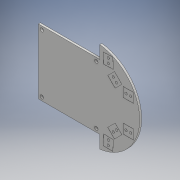
# Autodesk Inventor part: PCB_final
Saved by Autodesk Inventor 2017 (Build 210142000, 142)
## iProperties
Created: 2016-07-30
Part Number: PCB_final
Material: Generic
Document SubType Name: Modeling
Designer: ANDRES
Density: 1 g/cm^3
Appearance: Default
Author: ANDRES
Autodesk Inventor part; units mm, degrees
ref_plane "YZ Plane" through (0, 0, 0) normal (1, 0, 0) x (0, 1, 0)
ref_plane "XZ Plane" through (0, 0, 0) normal (0, 1, 0) x (-1, 0, 0)
ref_plane "XY Plane" through (0, 0, 0) normal (0, 0, 1) x (1, 0, 0)
sketch "Sketch1" plane through (0, 0, 0) normal (0, 1, 0) x (-1, 0, 0)
  circle A0 centre (-24.5, -25) radius 1.5
  circle A1 centre (-24.5, 25) radius 1.5
  circle A2 centre (22.5, 25) radius 1.5
  circle A3 centre (22.5, -25) radius 1.5
  line L0 (-27.5, -28) -> (-8, -28)
  line L1 (-8, -28) -> (-8, -25) construction
  line L2 (6, -25) -> (6, -28) construction
  line L3 (6, -28) -> (25.5, -28)
  line L4 (25.5, -28) -> (25.5, 28)
  line L5 (25.5, 28) -> (6, 28)
  line L6 (-8, 28) -> (-27.5, 28)
  line L7 (-27.5, 28) -> (-27.5, 39.1)
  arc A4 (-27.5, 39.1) -> (-27.5, -39.1) centre (-22.3277, 0) ccw
  line L8 (-27.5, -39.1) -> (-27.5, -28)
  line L9 (-8, 28) -> (6, 28)
  line L10 (-8, -25) -> (-8, 28) construction
  line L11 (6, -25) -> (6, 28) construction
  line L12 (-8, -28) -> (6, -28)
  line L13 (22.75, 28) -> (-24.75, 28) construction
  line L14 (-24.75, 22) -> (22.75, 22) construction
  line L15 (25.5, -22) -> (-24.75, -22) construction
  line L16 (-24.75, -28) -> (22.75, -28) construction
  line L17 (-8, 28) -> (-27.5, 28) construction
  line L18 (-27.5, 28) -> (-27.5, 39.1) construction
  arc A5 (-27.5, 39.1) -> (-27.5, -39.1) centre (-22.3277, 0) ccw construction
  circle A6 centre (-38.9568, 20.5358) radius 1
  line L19 (-40.0897, 25.2111) -> (-34.2841, 19.3919)
  line L20 (-46.4612, 18.8546) -> (-40.0897, 25.2111)
  circle A7 centre (-41.7885, 17.7107) radius 1
  line L21 (-46.4612, 18.8546) -> (-40.6556, 13.0354)
  line L22 (-34.2841, 19.3919) -> (-40.6556, 13.0354)
  line L23 (-39.9854, 35.3107) -> (-39.9038, 35.3078) construction
  circle A8 centre (-34.6947, 32.6244) radius 1
  line L24 (-39.0291, 26.2718) -> (-38.7163, 35.2301)
  circle A9 centre (-34.8343, 28.6268) radius 1
  line L25 (-39.0291, 26.2718) -> (-30.8141, 25.9849)
  line L26 (-30.5, 34.9794) -> (-30.8141, 25.9849)
  circle A10 centre (-50.0144, 13.6765) radius 1
  line L27 (-47.5144, 9.5665) -> (-47.5144, 17.7865)
  circle A11 centre (-54.0144, 13.6765) radius 1
  line L28 (-56.5144, 17.7865) -> (-47.5144, 17.7865)
  line L29 (-56.5144, 9.5665) -> (-56.5144, 17.7865)
  line L30 (-47.5144, 9.5665) -> (-56.5144, 9.5665)
  line L31 (-39.0291, 26.2718) -> (-67.0612, -1.7603) construction
  line L32 (-39.0291, 26.2718) -> (0.6143, 26.2718) construction
  line L33 (-38.7163, 35.2301) -> (-30.5, 34.9794)
  line L34 (-27.5, -28) -> (-27.5, -22) construction
  line L35 (-27.5, -22) -> (-24.75, -22) construction
  line L36 (-27.5, 28) -> (-27.5, 22) construction
  line L37 (-24.75, 22) -> (-27.5, 22) construction
  line L38 (-27.5, 22) -> (-27.5, 28) construction
  line L39 (-27.5, -22) -> (-27.5, -28) construction
  point P0 (0, 0)
  point P1 (0, 0)
  point P2 (-1, 28)
  point P3 (-1, -22)
  point P4 (-1, -28)
  point P5 (0, 0)
  point P6 (4.5, 0)
  dimension "d0" = 47.5
  dimension "d1" = 6
  dimension "d3" = 47.5
  dimension "d4" = 6
  dimension "d8" = 39.4406
  dimension "d9" = 5.1723
  dimension "d10" = 3
  dimension "d11" = 3
  dimension "d12" = 3
  dimension "d13" = 3
  dimension "d14" = 2
  dimension "d15" = 2
  dimension "d16" = 135
  dimension "d17" = 178
  dimension "d18" = 180
  dimension "d19" = 1.5
  dimension "d20" = 1.5
  dimension "d21" = 1.7282
  dimension "d22" = 8.22
  dimension "d23" = 9
  dimension "d24" = 2
  dimension "d25" = 2
  dimension "d26" = 2.5
  dimension "d27" = 4.11
  dimension "d28" = 4.11
  dimension "d29" = 2.5
  dimension "d30" = 8.22
  dimension "d31" = 2.5
  dimension "d32" = 9
  dimension "d33" = 2.5
  dimension "d34" = 4.11
  dimension "d35" = 4.11
  dimension "d36" = 9
  dimension "d37" = 8.22
  dimension "d38" = 4.11
  dimension "d39" = 2.5
  dimension "d40" = 2.5
  dimension "d41" = 4.11
  dimension "d42" = 3
  dimension "d58" = 3
  dimension "d59" = 53
  dimension "d60" = 3
  dimension "d61" = 3
  dimension "d62" = 3
  constraints: 80 end point, 12 centre point, 7 horizontal, 6 perpendicular, 5 point on circle, 5 point on line, 4 midpoint, 4 parallel, 2 collinear, 1 equal length, 1 vertical
  measures "d0" distance of L14.end L14.start
  measures "d1" distance of L14.start L13.end
  measures "d3" distance of L16.end L16.start
  measures "d4" distance of L16.start L15.end
  measures "d8" radius of A4
  measures "d9" distance from line of L8 A4.centre
  measures "d10" distance from line of L5 A2.centre
  measures "d11" distance from line of L6 A1.centre
  measures "d12" distance from line of L0 A0.centre
  measures "d13" distance from line of L3 A3.centre
  measures "d14" diameter of A9
  measures "d15" diameter of A8
  measures "d16" angle of L31 L32
  measures "d17" angle of L32 L25
  measures "d18" angle of L32 L30
  measures "d19" distance from line of L31.start L19
  measures "d20" distance from line of L27.end L21
  measures "d21" distance between parallel lines of L32 L17
  measures "d22" distance between parallel lines of L28 L30
  measures "d23" distance between parallel lines of L29 L27
  measures "d24" diameter of A11
  measures "d25" diameter of A10
  measures "d26" distance from line of L27 A10.centre
  measures "d27" distance from line of L30 A10.centre
  measures "d28" distance from line of L30 A11.centre
  measures "d29" distance from line of L29 A11.centre
  measures "d30" distance between parallel lines of L20 L22
  measures "d31" distance from line of L21 A7.centre
  measures "d32" distance between parallel lines of L19 L21
  measures "d33" distance from line of A6.centre L19
  measures "d34" distance from line of L22 A6.centre
  measures "d35" distance from line of L22 A7.centre
  measures "d36" distance between parallel lines of L23 L25
  measures "d37" distance between parallel lines of L26 L24
  measures "d38" distance from line of L24 A8.centre
  measures "d39" distance from line of L23 A8.centre
  measures "d40" distance from line of L25 A9.centre
  measures "d41" distance from line of L24 A9.centre
  measures "d42" distance from line of L18 L26.start
  measures "d58" distance from line of L4 A2.centre
  measures "d59" distance between parallel lines of L8 L4
  measures "d60" distance from line of L34 A0.centre
  measures "d61" distance from line of L36 A1.centre
  measures "d62" distance from line of A3.centre L4
extrude "Extrusion1" add sketch "Sketch1" along normal blind 1.75 contours L8 A4 L7 L6 L9 L5 L4 L3 L12 L0 | A6 | L19 L22 L21 L20 | A7 | A8 | L24 L33 L26 L25 | A9 | A10 | L30 L29 L28 L27 | A11
sketch "Sketch2" plane through (0, 0, 0) normal (0, -1, 0) x (1, 0, 0)
  circle A0 centre (-17.5, -25) radius 1.5
  circle A1 centre (-17.5, 25) radius 1.5
  circle A2 centre (19.5, 25) radius 1.5
  circle A3 centre (19.5, -25) radius 1.5
  line L0 (27.5, -28) -> (-25.5, -28) projected
  line L1 (27.5, -39.1) -> (27.5, -28) projected
  arc A4 (27.5, 39.1) -> (27.5, -39.1) centre (22.3277, 0) ccw projected
  line L2 (27.5, 28) -> (27.5, 39.1) projected
  line L3 (-25.5, 28) -> (27.5, 28) projected
  line L4 (-25.5, -28) -> (-25.5, 28) projected
  line L5 (24.75, 28) -> (-22.75, 28)
  line L6 (-22.75, 28) -> (-22.75, 22)
  line L7 (-22.75, 22) -> (24.75, 22)
  line L8 (24.75, 22) -> (24.75, 28)
  line L9 (24.75, -22) -> (-22.75, -22)
  line L10 (-22.75, -22) -> (-22.75, -28)
  line L11 (-22.75, -28) -> (24.75, -28)
  line L12 (24.75, -28) -> (24.75, -22)
  point P0 (0, 0)
  point P1 (1, 28)
  point P2 (1, -28)
  dimension "d45" = 47.5
  dimension "d46" = 6
  dimension "d48" = 5.25
  dimension "d49" = 5.25
  dimension "d50" = 47.5
  dimension "d51" = 6
  dimension "d52" = 5.25
  dimension "d53" = 5.25
  constraints: 16 end point, 8 centre point, 4 midpoint, 4 parallel, 2 horizontal, 2 perpendicular
  measures "d45" distance of L7.end L6.end
  measures "d46" distance of L6.end L5.end
  measures "d48" distance from line of L6 A1.centre
  measures "d49" distance from line of L8 A2.centre
  measures "d50" distance of L11.end L10.end
  measures "d51" distance of L10.end L9.end
  measures "d52" distance from line of L12 A3.centre
  measures "d53" distance from line of L10 A0.centre
extrude "Extrusion2" cut sketch "Sketch1" along normal blind 0.1 contours L19 L22 L21 L20 | L24 L33 L26 L25 | L30 L29 L28 L27
mirror "Mirror1" about plane through (0, 0, 0) normal (0, 0, 1) of "Extrusion2"
body "Solid1"
